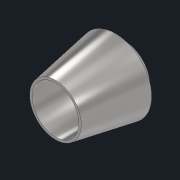
# Autodesk Inventor part: rod330_end_cap
Saved by Autodesk Inventor 2022 (Build 260153000, 153)
## iProperties
Created: 2024-03-31
Part Number: rod330_end_cap
Material: ステンレス鋼
Document SubType Name: Modeling
Designer: gisen
Mass: 65.69 g
Surface Area: 48.7585 cm^2
Volume: 8.21125 cm^3
Density: 8 g/cm^3
Appearance: 半つや出し
Author: gisen
Autodesk Inventor part; units mm, degrees
ref_plane "YZ Plane" through (0, 0, 0) normal (1, 0, 0) x (0, 1, 0)
ref_plane "XZ Plane" through (0, 0, 0) normal (0, 1, 0) x (-1, 0, 0)
ref_plane "XY Plane" through (0, 0, 0) normal (0, 0, 1) x (1, 0, 0)
sketch "スケッチ1" plane through (0, 0, 0) normal (1, 0, 0) x (0, 1, 0)
  line L0 (10.2, 20) -> (10.2, 0)
  line L1 (10.2, 0) -> (9, 0)
  line L2 (9, 0) -> (9, -10)
  line L3 (9, -10) -> (11.0175, -10)
  line L4 (11.0175, -10) -> (15.7845, -6)
  line L5 (15.7845, -6) -> (11.2, 20)
  line L6 (11.2, 20) -> (10.2, 20)
  line L7 (0, -16) -> (0, 26) projected
  point P0 (0, 0)
  dimension "d0" = 20
  dimension "d1" = 9
  dimension "d2" = 10
  dimension "d3" = 10.2
  dimension "d4" = 1
  dimension "d5" = 10
  dimension "d7" = 4
  dimension "d9" = 120
  constraints: 14 end point, 4 perpendicular, 1 horizontal alignment, 1 vertical
  measures "d0" distance between parallel lines of L1 L6
  measures "d1" distance from line of point (0, 0) L2
  measures "d2" distance of L1.end L2.end
  measures "d3" distance from line of point (0, 0) L0
  measures "d4" distance of L5.end L0.start
  measures "d5" angle of L0 L5
  measures "d7" vertical distance of L3.end L4.end
  measures "d9" angle of L4 L5
revolve "回転1" add sketch "スケッチ1" angle 360 about axis through (0, 0, -10) along (0, 0, 1)
thread "ねじ1" size "M18x2" class "6H" standard "ISO Metric profile" full length
